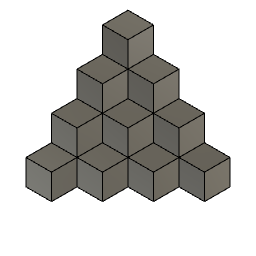
cube (Autodesk Fusion 360 design; units mm, degrees)
Autodesk Fusion 360 part; units mm, degrees
sketch "Sketch1" plane through (0, 0, 0) normal (0, 0, 1) x (1, 0, 0)
  line L0 (0, 0) -> (20, 0)
  line L1 (20, 0) -> (20, -80)
  line L2 (20, -80) -> (0, -80)
  line L3 (0, -80) -> (0, 0)
  line L4 (20, 0) -> (80, 0)
  line L5 (80, 0) -> (80, -20)
  line L6 (80, -20) -> (20, -20)
  line L7 (20, -20) -> (20, 0)
  line L8 (20, -20) -> (40, -20)
  line L9 (40, -20) -> (40, -60)
  line L10 (40, -60) -> (20, -60)
  line L11 (20, -60) -> (20, -20)
  line L12 (40, -20) -> (60, -20)
  line L13 (60, -20) -> (60, -40)
  line L14 (60, -40) -> (40, -40)
  line L15 (40, -40) -> (40, -20)
  dimension "d1" = 80
  dimension "d2" = 20
  dimension "d3" = 20
  dimension "d4" = 80
  dimension "d9" = 40
  dimension "d10" = 20
  dimension "d11" = 20
  dimension "d12" = 20
  constraint horizontal L0
  constraint vertical L1
  constraint horizontal L2
  constraint vertical L3
  constraint coincident L0.start L3.end
  constraint horizontal L4
  constraint vertical L5
  constraint horizontal L6
  constraint vertical L7
  constraint horizontal L8
  constraint vertical L9
  constraint horizontal L10
  constraint vertical L11
  constraint horizontal L12
  constraint vertical L13
  constraint horizontal L14
  constraint vertical L15
  measures "d1" distance of L0.end L1.end
  measures "d2" distance of L0.start L0.end
  measures "d3" distance of L4.end L5.end
  measures "d4" distance of L3 L5
  measures "d9" distance of L8.end L9.end
  measures "d10" distance of L9.end L10.end
  measures "d11" distance of L12.end L13.end
  measures "d12" distance of L13.end L14.end
extrude "Extrude2" add sketch "Sketch1" along normal blind 20 contours L0 L1 L2 L3 L7 L11 | L1 L4 L5 L6 L7 L8 L12
extrude "Extrude3" add sketch "Sketch1" along normal blind 20 contours L1 L6 L8 L9 L10 L11 L15 | L6 L9 L12 L13 L14 L15
sketch "Sketch2" plane through (0, 0, 20) normal (0, 0, 1) x (-1, 0, 0)
  line L0 (-80, 20) -> (-80, 0)
  line L1 (-80, 0) -> (0, 0)
  line L2 (0, 0) -> (0, 80)
  line L3 (0, 80) -> (-20, 80)
  line L4 (-20, 80) -> (-20, 60)
  line L5 (-20, 60) -> (-40, 60)
  line L6 (-40, 60) -> (-40, 40)
  line L7 (-40, 40) -> (-60, 40)
  line L8 (-60, 40) -> (-60, 20)
  line L9 (-60, 20) -> (-80, 20)
  line L10 (0, 0) -> (-20, 0)
  line L11 (-20, 0) -> (-20, 60)
  line L12 (-20, 60) -> (0, 60)
  line L13 (0, 60) -> (0, 0)
  line L14 (-20, 0) -> (-60, 0)
  line L15 (-60, 0) -> (-60, 20)
  line L16 (-60, 20) -> (-20, 20)
  line L17 (-20, 20) -> (-20, 0)
  line L18 (-20, 20) -> (-40, 20)
  line L19 (-40, 20) -> (-40, 40)
  line L20 (-40, 40) -> (-20, 40)
  line L21 (-20, 40) -> (-20, 20)
  constraint horizontal L10
  constraint vertical L11
  constraint horizontal L12
  constraint vertical L13
  constraint coincident L4.end L5.start
  constraint coincident L1.end L2.start
  constraint horizontal L14
  constraint vertical L15
  constraint horizontal L16
  constraint vertical L17
  constraint coincident L8.end L9.start
  constraint horizontal L18
  constraint vertical L19
  constraint horizontal L20
  constraint vertical L21
  constraint coincident L6.end L7.start
extrude "Extrude4" add sketch "Sketch2" along normal blind 20 contours L1 L11 L14 L15 L16 L17 L18 | L11 L16 L18 L19 L20 L21 | L1 L2 L10 L11 L12 L13 L17 L21
sketch "Sketch3" plane through (0, 0, 40) normal (0, 0, 1) x (-1, 0, 0)
  line L0 (-40, 40) -> (-40, 20)
  line L1 (-40, 20) -> (-60, 20)
  line L2 (-60, 20) -> (-60, 0)
  line L3 (-60, 0) -> (0, 0)
  line L4 (0, 0) -> (0, 60)
  line L5 (0, 60) -> (-20, 60)
  line L6 (-20, 60) -> (-20, 40)
  line L7 (-20, 40) -> (-40, 40)
  line L8 (0, 0) -> (-40, 0)
  line L9 (-40, 0) -> (-40, 20)
  line L10 (-40, 20) -> (0, 20)
  line L11 (0, 20) -> (0, 0)
  line L12 (0, 20) -> (-20, 20)
  line L13 (-20, 20) -> (-20, 40)
  line L14 (-20, 40) -> (0, 40)
  line L15 (0, 40) -> (0, 20)
  constraint horizontal L8
  constraint vertical L9
  constraint horizontal L10
  constraint vertical L11
  constraint coincident L0.end L1.start
  constraint coincident L3.end L4.start
  constraint horizontal L12
  constraint vertical L13
  constraint horizontal L14
  constraint vertical L15
  constraint coincident L6.end L7.start
extrude "Extrude5" add sketch "Sketch3" along normal blind 20 contours L3 L4 L8 L9 L10 L11 L12 | L4 L10 L12 L13 L14 L15
sketch "Sketch4" plane through (0, 0, 60) normal (0, 0, 1) x (-1, 0, 0)
  line L0 (0, 40) -> (-20, 40)
  line L1 (-20, 40) -> (-20, 20)
  line L2 (-20, 20) -> (-40, 20)
  line L3 (-40, 20) -> (-40, 0)
  line L4 (-40, 0) -> (0, 0)
  line L5 (0, 0) -> (0, 40)
  line L6 (0, 0) -> (-20, 0)
  line L7 (-20, 0) -> (-20, 20)
  line L8 (-20, 20) -> (0, 20)
  line L9 (0, 20) -> (0, 0)
  constraint horizontal L6
  constraint vertical L7
  constraint horizontal L8
  constraint vertical L9
  constraint coincident L1.end L2.start
  constraint coincident L4.end L5.start
extrude "Extrude6" add sketch "Sketch4" along normal blind 20 contours L4 L5 L6 L7 L8 L9
shell "Shell1" thickness 4 removed faces 1 at (20, -33.3333, 0)
